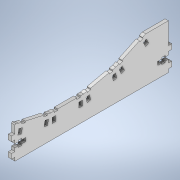
# Autodesk Inventor part: switchplate-support-06
Saved by Autodesk Inventor 2020.1 (Build 241239000, 239)
## iProperties
Created: 2019-06-27
Material: Acier, galvanisé
Document SubType Name: Modeling
Designer: Thibault
Density: 7.85 g/cm^3
Appearance: Aluminium - Poli
Mass: 11.7255 g
Surface Area: 33.7109 cm^2
Volume: 1.4937 cm^3
Part Number: switchplate-support-06
sa_0: 0.400 nd
height_shift: 0,000 mm
base_height: 27,000 mm
switchplate_depth: 121,000 mm
short_switchplate_depth: 96,296 mm
Author: Thibault
Autodesk Inventor part; units mm, degrees
ref_plane "YZ Plane" through (0, 0, 0) normal (1, 0, 0) x (0, 1, 0)
ref_plane "XZ Plane" through (0, 0, 0) normal (0, 1, 0) x (-1, 0, 0)
ref_plane "XY Plane" through (0, 0, 0) normal (0, 0, 1) x (1, 0, 0)
sketch "Anchor (screw side)" plane through (0, 0, 0) normal (0, 0, 1) x (1, 0, 0)
  circle A0 centre (93.8994, 50.3042) radius 1.05
  line L0 (90.8494, 51.3542) -> (87.7494, 51.3542)
  line L1 (87.7494, 51.3542) -> (87.7494, 49.2542)
  line L2 (87.7494, 49.2542) -> (90.8494, 49.2542)
  line L3 (90.8494, 49.2542) -> (90.8494, 51.3542)
  line L4 (100.0494, 51.3542) -> (96.9494, 51.3542)
  line L5 (96.9494, 51.3542) -> (96.9494, 49.2542)
  line L6 (96.9494, 49.2542) -> (100.0494, 49.2542)
  line L7 (100.0494, 49.2542) -> (100.0494, 51.3542)
  line L8 (90.8494, 51.3542) -> (96.9494, 49.2542) construction
  line L9 (96.9494, 51.3542) -> (90.8494, 49.2542) construction
  line L10 (85.7494, 53.3542) -> (102.0494, 53.3542) construction
  line L11 (102.0494, 53.3542) -> (102.0494, 47.2542) construction
  line L12 (102.0494, 47.2542) -> (85.7494, 47.2542) construction
  line L13 (85.7494, 47.2542) -> (85.7494, 53.3542) construction
  point P0 (103.5798, 50.1132)
  dimension "d27_1" = 2.1
  dimension "d28_1" = 3.1
  dimension "d29" = 2.1
  dimension "slot_distance" = 6.1
  dimension "d34" = 2
  dimension "d35" = 2
  dimension "d36" = 2
  dimension "d37" = 2
  measures "d27_1" diameter of A0
  measures "d28_1" distance of L2.end L1.end
  measures "d29" distance of L1.end L0.end
  measures "slot_distance" distance between parallel lines of L5 L3
  measures "d34" distance between parallel lines of L0 L10
  measures "d35" distance between parallel lines of L12 L2
  measures "d36" distance between parallel lines of L11 L7
  measures "d37" distance between parallel lines of L13 L1
sketch "Anchor (nut side)" plane through (0, 0, 0) normal (0, 0, 1) x (1, 0, 0)
  line L0 (11.1, 0) -> (9.1, 0)
  line L1 (9.1, 0) -> (9.1, -2)
  line L2 (9.1, -2) -> (9.9, -2)
  line L3 (9.9, -2) -> (9.9, -4)
  line L4 (6.2, -4) -> (6.2, -2)
  line L5 (6.2, -2) -> (7, -2)
  line L6 (7, -2) -> (7, 0)
  line L7 (7, 0) -> (5, 0)
  line L8 (2, 0) -> (2, 2)
  line L9 (2, 0) -> (3, 0) construction
  line L10 (2, 2) -> (5, 2)
  line L11 (5, 2) -> (5, 0)
  line L12 (11.1, 0) -> (11.1, 2)
  line L13 (11.1, 2) -> (14.1, 2)
  line L14 (14.1, 2) -> (14.1, 0)
  line L15 (0, 0) -> (2, 0)
  line L16 (14.1, 0) -> (16.1, 0)
  line L17 (6.2, -4) -> (7, -4)
  line L18 (9.9, -4) -> (9.1, -4)
  line L19 (7, -4) -> (7, -6.25)
  line L20 (9.1, -4) -> (9.1, -6.25)
  line L21 (7.25, -6.5) -> (8.05, -6.5)
  arc A0 (7, -6.25) -> (7.25, -6.5) centre (7.25, -6.25) ccw
  arc A1 (8.85, -6.5) -> (9.1, -6.25) centre (8.85, -6.25) ccw
  line L22 (8.05, -6.5) -> (8.85, -6.5)
  line L23 (8.05, -3.8983) -> (8.05, -9.959) construction
  point P0 (9.1321, -0.6227)
  point P1 (7, -6.5)
  point P2 (9.1, -6.5)
  dimension "d3" = 2
  dimension "d7" = 6.1
  dimension "d10" = 2
  dimension "d11" = 2
  dimension "d12" = 0.8
  dimension "d13" = 2
  dimension "d14" = 0.8
  dimension "d15" = 2.1
  dimension "d18" = 2
  dimension "d19" = 0.8
  dimension "d20" = 0.8
  dimension "d21" = 2.5
  dimension "d22" = 2.5
  dimension "d23" = 2.1
  dimension "d38" = 2
  dimension "d39" = 0.25
  dimension "d120" = 3
  measures "d3" distance of point (0, 0) L8.start
  measures "d7" distance of L7.end L0.start
  measures "d10" distance of L0.start L0.end
  measures "d11" distance of L0.end L1.end
  measures "d12" distance of L1.end L2.end
  measures "d13" distance of L2.end L3.end
  measures "d14" distance of L4.end L5.end
  measures "d15" distance of L6.end L0.end
  measures "d18" distance of L14.end point (16.1, 0)
  measures "d19" distance of L4.start L17.end
  measures "d20" distance of L3.end L18.end
  measures "d21" distance of L17.end point (7, -6.5)
  measures "d22" distance of L18.end point (9.1, -6.5)
  measures "d23" distance of L17.end L18.end
  measures "d38" distance of the line from the sketch origin of L10
  measures "d39" radius of A0
  measures "d120" distance of L8.end L10.end
sketch "Anchor (to 2ndary key support)" plane through (0, 0, 0) normal (0, 0, 1) x (1, 0, 0)
  line L0 (12.2429, 14.9506) -> (13.2929, 14.9506)
  line L1 (14.3429, 14.9506) -> (14.3429, 11.8506)
  line L2 (14.3429, 11.8506) -> (12.2429, 11.8506)
  line L3 (12.2429, 11.8506) -> (12.2429, 14.9506)
  line L4 (13.2929, 14.9506) -> (13.2929, 11.8506) construction
  line L5 (13.2929, 14.9506) -> (14.3429, 14.9506)
  point P0 (14.0267, 11.8837)
  dimension "d40" = 2.1
  dimension "d41" = 3.1
  measures "d40" distance of L1.end L2.end
  measures "d41" distance of L1.start L1.end
sketch "Switch support" plane through (0, 0, 0) normal (0, 0, 1) x (1, 0, 0)
  line L0 (14.375, 16.4474) -> (15.075, 16.4474)
  line L1 (15.075, 16.4474) -> (15.075, 15.6474)
  line L2 (15.075, 15.6474) -> (17.075, 15.6474)
  line L3 (17.075, 15.6474) -> (17.075, 16.4474)
  line L4 (17.075, 16.4474) -> (22.875, 16.4474)
  line L5 (28.675, 16.4474) -> (28.675, 15.6474)
  line L6 (28.675, 15.6474) -> (30.675, 15.6474)
  line L7 (30.675, 15.6474) -> (30.675, 16.4474)
  line L8 (30.675, 16.4474) -> (31.375, 16.4474)
  line L9 (22.875, 19.1721) -> (22.875, 15.8971) construction
  line L10 (22.875, 16.4474) -> (28.675, 16.4474)
  line L11 (13.775, 13.6474) -> (14.825, 13.6474)
  line L12 (15.875, 13.6474) -> (15.875, 10.5474)
  line L13 (15.875, 10.5474) -> (13.775, 10.5474)
  line L14 (13.775, 10.5474) -> (13.775, 13.6474)
  line L15 (14.825, 13.6474) -> (14.825, 10.5474) construction
  line L16 (14.825, 13.6474) -> (15.875, 13.6474)
  line L17 (29.875, 13.6474) -> (30.925, 13.6474)
  line L18 (31.975, 13.6474) -> (31.975, 10.5474)
  line L19 (31.975, 10.5474) -> (29.875, 10.5474)
  line L20 (29.875, 10.5474) -> (29.875, 13.6474)
  line L21 (30.925, 13.6474) -> (30.925, 10.5474) construction
  line L22 (30.925, 13.6474) -> (31.975, 13.6474)
  point P0 (20.0288, 26.7181)
  dimension "d43" = 0.8
  dimension "d44" = 2
  dimension "d45" = 11.6
  dimension "d46" = 2
  dimension "d47" = 0.7
  dimension "d48" = 17
  dimension "d51" = 2
  dimension "d121" = 8.05
  dimension "d123" = 8.05
  measures "d43" distance of L1.start L1.end
  measures "d44" distance of L1.end L2.end
  measures "d45" distance of L5.start L3.end
  measures "d46" distance of L5.end L6.end
  measures "d47" distance of L7.end point (31.375, 16.447)
  measures "d48" distance of point (31.375, 16.447) point (14.375, 16.447)
  measures "d51" length of L2
sketch "Sketch1" plane through (0, 0, 0) normal (1, 0, 0) x (0, 1, 0)
  line L0 (0, -121) -> (27, -121)
  line L1 (27, 0) -> (0, 0)
  line L2 (27, -121) -> (27, -105.3511)
  line L3 (26.5066, -12.0581) -> (27, -11)
  line L4 (28.2121, -16.9724) -> (22.1003, -16.9724)
  line L5 (26.4083, -12.2688) -> (27, -11)
  line L6 (19.2238, -27.6761) -> (18.6322, -28.9449)
  line L7 (21.9473, -35.6102) -> (15.8356, -35.6102)
  line L8 (18.3291, -30.3117) -> (18.6322, -28.9449)
  line L9 (14.6497, -46.9087) -> (14.3467, -48.2756)
  line L10 (19.8511, -55.1756) -> (13.7394, -55.1756)
  line L11 (14.3467, -49.6756) -> (14.3467, -48.2756)
  line L12 (14.3467, -66.6756) -> (14.3467, -68.0756)
  line L13 (22.0358, -74.7409) -> (15.9241, -74.7409)
  line L14 (14.6497, -69.4424) -> (14.3467, -68.0756)
  line L15 (18.3291, -86.0394) -> (18.6322, -87.4062)
  line L16 (28.3566, -93.3787) -> (22.2449, -93.3787)
  line L17 (19.2238, -88.675) -> (18.6322, -87.4062)
  line L18 (26.4083, -104.0823) -> (27, -105.3511)
  line L19 (27, 0) -> (27, -11)
  line L20 (0, 0) -> (0, -121)
  line L21 (18.3291, -30.3117) -> (18.1776, -30.9951)
  line L22 (18.1776, -30.9951) -> (17.3966, -30.822)
  line L23 (17.3966, -30.822) -> (16.9637, -32.7746)
  line L24 (16.9637, -32.7746) -> (17.7448, -32.9477)
  line L25 (17.7448, -32.9477) -> (16.4894, -38.6102)
  line L26 (15.2341, -44.2727) -> (14.453, -44.0996)
  line L27 (14.453, -44.0996) -> (14.0201, -46.0522)
  line L28 (14.0201, -46.0522) -> (14.8012, -46.2253)
  line L29 (14.8012, -46.2253) -> (14.6497, -46.9087)
  line L30 (19.1495, -39.2) -> (15.9521, -38.4911) construction
  line L31 (16.4894, -38.6102) -> (15.2341, -44.2727)
  line L32 (15.7254, -29.1199) -> (15.4981, -30.145)
  line L33 (15.2709, -31.1701) -> (12.2443, -30.4992)
  line L34 (12.2443, -30.4992) -> (12.6989, -28.4489)
  line L35 (12.6989, -28.4489) -> (15.7254, -29.1199)
  line L36 (15.4981, -30.145) -> (12.4716, -29.474) construction
  line L37 (15.4981, -30.145) -> (15.2709, -31.1701)
  line L38 (12.2407, -44.8383) -> (12.0134, -45.8634)
  line L39 (11.7862, -46.8885) -> (8.7597, -46.2175)
  line L40 (8.7597, -46.2175) -> (9.2142, -44.1673)
  line L41 (9.2142, -44.1673) -> (12.2407, -44.8383)
  line L42 (12.0134, -45.8634) -> (8.9869, -45.1924) construction
  line L43 (12.0134, -45.8634) -> (11.7862, -46.8885)
  line L44 (26.4083, -12.2688) -> (26.1125, -12.9032)
  line L45 (26.1125, -12.9032) -> (25.3875, -12.5652)
  line L46 (25.3875, -12.5652) -> (24.5422, -14.3778)
  line L47 (24.5422, -14.3778) -> (25.2673, -14.7159)
  line L48 (25.2673, -14.7159) -> (22.8161, -19.9724)
  line L49 (20.3649, -25.229) -> (19.6398, -24.8909)
  line L50 (19.6398, -24.8909) -> (18.7946, -26.7036)
  line L51 (18.7946, -26.7036) -> (19.5197, -27.0416)
  line L52 (19.5197, -27.0416) -> (19.2238, -27.6761)
  line L53 (25.2855, -21.1239) -> (22.3173, -19.7399) construction
  line L54 (22.8161, -19.9724) -> (20.3649, -25.229)
  line L55 (24.1242, -10.5417) -> (23.6805, -11.4933)
  line L56 (23.2367, -12.445) -> (20.4272, -11.1348)
  line L57 (20.4272, -11.1348) -> (21.3147, -9.2316)
  line L58 (21.3147, -9.2316) -> (24.1242, -10.5417)
  line L59 (23.6805, -11.4933) -> (20.8709, -10.1832) construction
  line L60 (23.6805, -11.4933) -> (23.2367, -12.445)
  line L61 (17.3201, -25.1333) -> (16.8763, -26.0849)
  line L62 (16.4326, -27.0365) -> (13.623, -25.7264)
  line L63 (13.623, -25.7264) -> (14.5105, -23.8232)
  line L64 (14.5105, -23.8232) -> (17.3201, -25.1333)
  line L65 (16.8763, -26.0849) -> (14.0668, -24.7748) construction
  line L66 (16.8763, -26.0849) -> (16.4326, -27.0365)
  line L67 (14.3467, -49.6756) -> (14.3467, -50.3756)
  line L68 (14.3467, -50.3756) -> (13.5467, -50.3756)
  line L69 (13.5467, -50.3756) -> (13.5467, -52.3756)
  line L70 (13.5467, -52.3756) -> (14.3467, -52.3756)
  line L71 (14.3467, -52.3756) -> (14.3467, -58.1756)
  line L72 (14.3467, -63.9756) -> (13.5467, -63.9756)
  line L73 (13.5467, -63.9756) -> (13.5467, -65.9756)
  line L74 (13.5467, -65.9756) -> (14.3467, -65.9756)
  line L75 (14.3467, -65.9756) -> (14.3467, -66.6756)
  line L76 (17.0713, -58.1756) -> (13.7963, -58.1756) construction
  line L77 (14.3467, -58.1756) -> (14.3467, -63.9756)
  line L78 (11.5467, -49.0756) -> (11.5467, -50.1256)
  line L79 (11.5467, -51.1756) -> (8.4467, -51.1756)
  line L80 (8.4467, -51.1756) -> (8.4467, -49.0756)
  line L81 (8.4467, -49.0756) -> (11.5467, -49.0756)
  line L82 (11.5467, -50.1256) -> (8.4467, -50.1256) construction
  line L83 (11.5467, -50.1256) -> (11.5467, -51.1756)
  line L84 (11.5467, -65.1756) -> (11.5467, -66.2256)
  line L85 (11.5467, -67.2756) -> (8.4467, -67.2756)
  line L86 (8.4467, -67.2756) -> (8.4467, -65.1756)
  line L87 (8.4467, -65.1756) -> (11.5467, -65.1756)
  line L88 (11.5467, -66.2256) -> (8.4467, -66.2256) construction
  line L89 (11.5467, -66.2256) -> (11.5467, -67.2756)
  line L90 (14.6497, -69.4424) -> (14.8012, -70.1258)
  line L91 (14.8012, -70.1258) -> (14.0201, -70.2989)
  line L92 (14.0201, -70.2989) -> (14.453, -72.2515)
  line L93 (14.453, -72.2515) -> (15.2341, -72.0784)
  line L94 (15.2341, -72.0784) -> (16.4894, -77.7409)
  line L95 (17.7448, -83.4034) -> (16.9637, -83.5766)
  line L96 (16.9637, -83.5766) -> (17.3966, -85.5291)
  line L97 (17.3966, -85.5291) -> (18.1776, -85.356)
  line L98 (18.1776, -85.356) -> (18.3291, -86.0394)
  line L99 (19.1495, -77.1512) -> (15.9521, -77.86) construction
  line L100 (16.4894, -77.7409) -> (17.7448, -83.4034)
  line L101 (11.7862, -69.4626) -> (12.0134, -70.4877)
  line L102 (12.2407, -71.5128) -> (9.2142, -72.1838)
  line L103 (9.2142, -72.1838) -> (8.7597, -70.1336)
  line L104 (8.7597, -70.1336) -> (11.7862, -69.4626)
  line L105 (12.0134, -70.4877) -> (8.9869, -71.1587) construction
  line L106 (12.0134, -70.4877) -> (12.2407, -71.5128)
  line L107 (15.2709, -85.181) -> (15.4981, -86.2061)
  line L108 (15.7254, -87.2312) -> (12.6989, -87.9022)
  line L109 (12.6989, -87.9022) -> (12.2443, -85.852)
  line L110 (12.2443, -85.852) -> (15.2709, -85.181)
  line L111 (15.4981, -86.2061) -> (12.4716, -86.8771) construction
  line L112 (15.4981, -86.2061) -> (15.7254, -87.2312)
  line L113 (19.2238, -88.675) -> (19.5197, -89.3095)
  line L114 (19.5197, -89.3095) -> (18.7946, -89.6476)
  line L115 (18.7946, -89.6476) -> (19.6398, -91.4602)
  line L116 (19.6398, -91.4602) -> (20.3649, -91.1221)
  line L117 (20.3649, -91.1221) -> (22.8161, -96.3787)
  line L118 (25.2673, -101.6352) -> (24.5422, -101.9733)
  line L119 (24.5422, -101.9733) -> (25.3875, -103.786)
  line L120 (25.3875, -103.786) -> (26.1125, -103.4479)
  line L121 (26.1125, -103.4479) -> (26.4083, -104.0823)
  line L122 (25.2855, -95.2272) -> (22.3173, -96.6112) construction
  line L123 (22.8161, -96.3787) -> (25.2673, -101.6352)
  line L124 (16.4326, -89.3146) -> (16.8763, -90.2662)
  line L125 (17.3201, -91.2178) -> (14.5105, -92.528)
  line L126 (14.5105, -92.528) -> (13.623, -90.6247)
  line L127 (13.623, -90.6247) -> (16.4326, -89.3146)
  line L128 (16.8763, -90.2662) -> (14.0668, -91.5763) construction
  line L129 (16.8763, -90.2662) -> (17.3201, -91.2178)
  line L130 (23.2367, -103.9061) -> (23.6805, -104.8578)
  line L131 (24.1242, -105.8094) -> (21.3147, -107.1195)
  line L132 (21.3147, -107.1195) -> (20.4272, -105.2163)
  line L133 (20.4272, -105.2163) -> (23.2367, -103.9061)
  line L134 (23.6805, -104.8578) -> (20.8709, -106.1679) construction
  line L135 (23.6805, -104.8578) -> (24.1242, -105.8094)
  point P0 (19.2238, -88.675)
  point P1 (18.3291, -86.0394)
  point P2 (14.6497, -69.4424)
  point P3 (14.3467, -49.6756)
  point P4 (14.6497, -46.9087)
  point P5 (19.2238, -27.6761)
  point P6 (26.4083, -12.2688)
  dimension "height" = 27
  dimension "d193" = 27
  dimension "k1_a" = 1.4
  dimension "k1_b" = 1.4
  dimension "k2_a" = 1.4
  dimension "k2_b" = 1.4
  dimension "k3_a" = 1.4
  dimension "k3_b" = 1.4
  dimension "k4_a" = 1.4
  dimension "k4_b" = 1.4
  dimension "k5_a" = 1.4
  dimension "k5_b" = 1.4
  dimension "d257" = 11
  dimension "k1_angle" = 115
  dimension "k2_angle" = 102.5
  dimension "k3_angle" = 90
  dimension "k4_angle" = 77.5
  dimension "k5_angle" = 65
  constraints: 42 end point, 7 horizontal, 4 vertical, 1 collinear, 1 vertical alignment, 19 other
  measures "height" distance of L1.start L1.end
  measures "d193" distance of L0.end L0.start
  measures "k1_a" distance of L3.end L5.start
  measures "k1_b" distance of L6.end L6.start
  measures "k2_a" distance of L8.start L6.end
  measures "k2_b" distance of L9.end L9.start
  measures "k3_a" distance of L11.start L9.end
  measures "k3_b" distance of L12.end L12.start
  measures "k4_a" distance of L14.start L12.end
  measures "k4_b" distance of L15.end L15.start
  measures "k5_a" distance of L17.start L15.end
  measures "k5_b" distance of L2.end L18.start
  measures "d257" distance of L1.start L3.end
  measures "k3_angle" angle to the sketch y axis of L10
extrude "Base" add sketch "Sketch1" along normal blind 2
sketch "Sketch2" plane through (0, 0, 0) normal (-1, 0, 0) x (0, 0, 1)
  line L0 (-190.1228, 20.337) -> (-190.1228, -18.1383)
  line L1 (129.0949, 104.0572) -> (129.0949, -18.1383)
  line L2 (129.0949, -18.1383) -> (-190.1228, -18.1383)
  line L3 (-121, 0) -> (-121, 0) construction
  line L4 (-119, 16.1) -> (-119, 104.9044)
  line L5 (-119, 104.9044) -> (-190.1228, 104.9044)
  line L6 (-190.1228, 104.9044) -> (-190.1228, 20.337)
  line L7 (-2, 16.1) -> (-2, 104.0572)
  line L8 (-2, 104.0572) -> (129.0949, 104.0572)
  line L9 (0, 27) -> (0, 0) projected
  line L10 (-121, 0) -> (-121, 27) projected
  line L11 (0, 0) -> (-121, 0) projected
  line L12 (-2, 0) -> (-119, 0)
  line L13 (-119, 11.1) -> (-119, 9.1)
  line L14 (-119, 9.1) -> (-117, 9.1)
  line L15 (-117, 9.1) -> (-117, 9.9)
  line L16 (-117, 9.9) -> (-115, 9.9)
  line L17 (-115, 6.2) -> (-117, 6.2)
  line L18 (-117, 6.2) -> (-117, 7)
  line L19 (-117, 7) -> (-119, 7)
  line L20 (-119, 7) -> (-119, 5)
  line L21 (-119, 2) -> (-121, 2)
  line L22 (-119, 2) -> (-119, 3) construction
  line L23 (-121, 2) -> (-121, 5)
  line L24 (-121, 5) -> (-119, 5)
  line L25 (-119, 11.1) -> (-121, 11.1)
  line L26 (-121, 11.1) -> (-121, 14.1)
  line L27 (-121, 14.1) -> (-119, 14.1)
  line L28 (-119, 0) -> (-119, 2)
  line L29 (-119, 14.1) -> (-119, 16.1)
  line L30 (-115, 6.2) -> (-115, 7)
  line L31 (-115, 9.9) -> (-115, 9.1)
  line L32 (-115, 7) -> (-112.75, 7)
  line L33 (-115, 9.1) -> (-112.75, 9.1)
  line L34 (-112.5, 7.25) -> (-112.5, 8.05)
  arc A0 (-112.75, 7) -> (-112.5, 7.25) centre (-112.75, 7.25) ccw
  arc A1 (-112.5, 8.85) -> (-112.75, 9.1) centre (-112.75, 8.85) ccw
  line L35 (-112.5, 8.05) -> (-112.5, 8.85)
  line L36 (-115.1017, 8.05) -> (-109.041, 8.05) construction
  line L37 (-2, 5) -> (-2, 7)
  line L38 (-2, 7) -> (-4, 7)
  line L39 (-4, 7) -> (-4, 6.2)
  line L40 (-4, 6.2) -> (-6, 6.2)
  line L41 (-6, 9.9) -> (-4, 9.9)
  line L42 (-4, 9.9) -> (-4, 9.1)
  line L43 (-4, 9.1) -> (-2, 9.1)
  line L44 (-2, 9.1) -> (-2, 11.1)
  line L45 (-2, 14.1) -> (0, 14.1)
  line L46 (-2, 14.1) -> (-2, 13.1) construction
  line L47 (0, 14.1) -> (0, 11.1)
  line L48 (0, 11.1) -> (-2, 11.1)
  line L49 (-2, 5) -> (0, 5)
  line L50 (0, 5) -> (0, 2)
  line L51 (0, 2) -> (-2, 2)
  line L52 (-2, 16.1) -> (-2, 14.1)
  line L53 (-2, 2) -> (-2, 0)
  line L54 (-6, 9.9) -> (-6, 9.1)
  line L55 (-6, 6.2) -> (-6, 7)
  line L56 (-6, 9.1) -> (-8.25, 9.1)
  line L57 (-6, 7) -> (-8.25, 7)
  line L58 (-8.5, 8.85) -> (-8.5, 8.05)
  arc A2 (-8.25, 9.1) -> (-8.5, 8.85) centre (-8.25, 8.85) ccw
  arc A3 (-8.5, 7.25) -> (-8.25, 7) centre (-8.25, 7.25) ccw
  line L59 (-8.5, 8.05) -> (-8.5, 7.25)
  line L60 (-5.8983, 8.05) -> (-11.959, 8.05) construction
  point P0 (-119, 16.1)
  point P1 (-2, 16.1)
  point P2 (-2, 0)
  constraints: 20 end point, 4 vertical, 3 horizontal, 2 parallel, 1 perpendicular, 4 other
extrude "Standard anchors" cut sketch "Sketch2" against normal through all
sketch "Esquisse7" plane through (0, 0, 0) normal (-1, 0, 0) x (0, 0, 1)
  line L0 (-104.5, 8.35) -> (-102.5, 8.35) construction
  line L1 (-106.5, 9.15) -> (-104.5, 9.15) construction
  line L2 (-104.5, 5.85) -> (-106.5, 5.85) construction
  line L3 (-102.5, 6.65) -> (-104.5, 6.65) construction
  line L4 (-109, 9.15) -> (-100.5, 9.15)
  line L5 (-109, 5.85) -> (-100.5, 5.85)
  line L6 (-109, 10) -> (-109, 8.35) construction
  line L7 (-109, 9.15) -> (-109, 5.85)
  arc A0 (-102.5, 6.65) -> (-102.5, 8.35) centre (-102.5, 7.5) ccw projected
  line L8 (-100.5, 5.85) -> (-100.5, 9.15)
  point P0 (1.5, 20)
  point P1 (108.5, 20)
  point P2 (108.5, 0)
  point P3 (1.5, 0)
  point P4 (-2, 10)
  point P5 (-2, 5)
  point P6 (7.6691, 10.85)
  point P7 (8.8147, 9.7576)
  point P8 (-111, 0)
  point P9 (-102.77, 8.35)
  point P10 (-100.7609, 7.9198)
  dimension "d203" = 2
  constraints: 8 end point, 2 collinear, 1 perpendicular, 1 vertical, 2 other
  measures "d203" distance from line of L8 A0.centre
extrude "No back screw hole" [suppressed]
sketch "Esquisse13" plane through (2, 0, 0) normal (1, 0, 0) x (0, 0, -1)
  line L0 (23.8232, 14.5105) -> (25.1333, 17.3201)
  line L1 (25.1333, 17.3201) -> (27.0365, 16.4326)
  line L2 (27.0365, 16.4326) -> (25.7264, 13.623)
  line L3 (25.7264, 13.623) -> (23.8232, 14.5105)
  line L4 (27.0365, 16.4326) -> (25.7264, 13.623) projected
  line L5 (23.8232, 14.5105) -> (25.1333, 17.3201) projected
  line L6 (25.1333, 17.3201) -> (27.0365, 16.4326) projected
  line L7 (25.7264, 13.623) -> (23.8232, 14.5105) projected
  point P0 (0, 0)
  constraints: 8 end point, 4 collinear
extrude "Hole fixup" add sketch "Esquisse13" against normal blind 2
sketch "Esquisse8" plane through (0, 0, 0) normal (-1, 0, 0) x (0, 0, 1)
  line L0 (0, 0) -> (-100.5509, 0) projected
  line L1 (0, 0) -> (-20.4545, 0)
  line L2 (0, 67.271) -> (0, 0)
  line L3 (0, 27) -> (0, 0) projected
  line L4 (-26.7036, 67.271) -> (0, 67.271)
  line L5 (-26.7036, 67.271) -> (-26.7036, 16.1)
  line L6 (-121, 2) -> (-121, 27) projected
  line L7 (-26.7036, 5) -> (-26.7036, 7)
  line L8 (-26.7036, 7) -> (-28.7036, 7)
  line L9 (-28.7036, 7) -> (-28.7036, 6.2)
  line L10 (-28.7036, 6.2) -> (-30.7036, 6.2)
  line L11 (-30.7036, 9.9) -> (-28.7036, 9.9)
  line L12 (-28.7036, 9.9) -> (-28.7036, 9.1)
  line L13 (-28.7036, 9.1) -> (-26.7036, 9.1)
  line L14 (-26.7036, 9.1) -> (-26.7036, 11.1)
  line L15 (-26.7036, 14.1) -> (-24.7036, 14.1)
  line L16 (-26.7036, 14.1) -> (-26.7036, 13.1) construction
  line L17 (-24.7036, 14.1) -> (-24.7036, 11.1)
  line L18 (-24.7036, 11.1) -> (-26.7036, 11.1)
  line L19 (-26.7036, 5) -> (-24.7036, 5)
  line L20 (-24.7036, 5) -> (-24.7036, 2)
  line L21 (-24.7036, 2) -> (-26.7036, 2)
  line L22 (-26.7036, 16.1) -> (-26.7036, 14.1)
  line L23 (-26.7036, 2) -> (-26.7036, 0)
  line L24 (-30.7036, 9.9) -> (-30.7036, 9.1)
  line L25 (-30.7036, 6.2) -> (-30.7036, 7)
  line L26 (-30.7036, 9.1) -> (-32.9536, 9.1)
  line L27 (-30.7036, 7) -> (-32.9536, 7)
  line L28 (-33.2036, 8.85) -> (-33.2036, 8.05)
  arc A0 (-32.9536, 9.1) -> (-33.2036, 8.85) centre (-32.9536, 8.85) ccw
  arc A1 (-33.2036, 7.25) -> (-32.9536, 7) centre (-32.9536, 7.25) ccw
  line L29 (-33.2036, 8.05) -> (-33.2036, 7.25)
  line L30 (-30.6018, 8.05) -> (-36.6626, 8.05) construction
  point P0 (110, 0)
  point P1 (-109, 0)
  point P2 (-121, 0)
  point P3 (0, 12.75)
  point P4 (0, 10.25)
  point P5 (0, 12)
  point P6 (-26.7036, 0)
  point P7 (-121, 5)
  point P8 (-26.7036, 18.7946)
  dimension "d232" = 20.4545
  constraints: 8 end point, 3 vertical, 2 collinear, 2 horizontal, 1 parallel, 1 point on line, 1 other
  measures "d232" distance of L0.start L1.end
extrude "Short plate" cut sketch "Esquisse8" against normal through all
derived "shared_parameters.ipt"
equation "\"depth_shift\" = 5"
equation "\"angle\" = 12.5deg"
equation "\"a_default\" = 1.4"
equation "\"b_default\" = 1.4"
